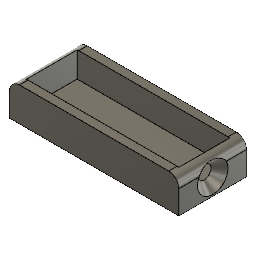
ANNE (Autodesk Fusion 360 design; units mm, degrees)
Autodesk Fusion 360 part; units mm, degrees
sketch "Sketch1" plane through (0, 0, 0) normal (0, 1, 0) x (1, 0, 0)
  line L0 (50, 20) -> (-50, 20)
  line L1 (-50, 20) -> (-50, -20)
  line L2 (-50, -20) -> (50, -20)
  line L3 (50, -20) -> (50, 20)
  line L4 (50, 20) -> (-50, -20) construction
  line L5 (-50, 20) -> (50, -20) construction
  dimension "d7" = 100
  dimension "d8" = 40
  constraint horizontal L0
  constraint perpendicular L0 L1
  constraint parallel L0 L2
  constraint parallel L1 L3
  constraint coincident L4 origin
  constraint coincident L5 origin
  measures "d7" distance of L1.end L2.end
  measures "d8" distance of L0.end L1.end
extrude "Extrude1" add sketch "Sketch1" along normal blind 20
shell "Shell1" thickness 5 removed faces 1 at (-16.6667, 20, -6.6667)
sketch "Sketch2" plane through (50, 0, 0) normal (1, 0, 0) x (0, 0, -1)
  line L0 (-20, 0) -> (20, 0)
  line L1 (20, 0) -> (20, 20)
  line L2 (20, 20) -> (-20, 20)
  line L3 (-20, 20) -> (-20, 0)
  circle A0 centre (0, 10) radius 4
  dimension "d12" = 8
  measures "d12" diameter of A0
extrude "Extrude2" cut sketch "Sketch2" against normal blind 5 contours A0
chamfer "Chamfer1" distance 5 angle 45 1 edges at (50, 11.4465, 3.7293)
fillet "Fillet1" radius 6 1 edges at (-50, 20, 0)
fillet "Fillet2" radius 6 1 edges at (50, 20, 0)
equation "length = 100 mm" comment "user parameter"
equation "width = length * 0.4" comment "useer parameter"
equation "height = width / 2" comment "user parameter"
equation "wallthickness = 5 mm" comment "user paremeter"
equation "holesize = 8 mm" comment "user parameter"
equation "chamfer = 5 mm" comment "user parameter"
equation "d7 = length"
equation "d8 = width"
equation "d9 = height"
equation "d11 = wallthickness"
equation "d12 = holesize"
equation "d13 = -wallthickness"
equation "d15 = chamfer"
equation "fillet = 6 mm" comment "user parameter"
equation "d17 = fillet"
equation "d18 = fillet"
